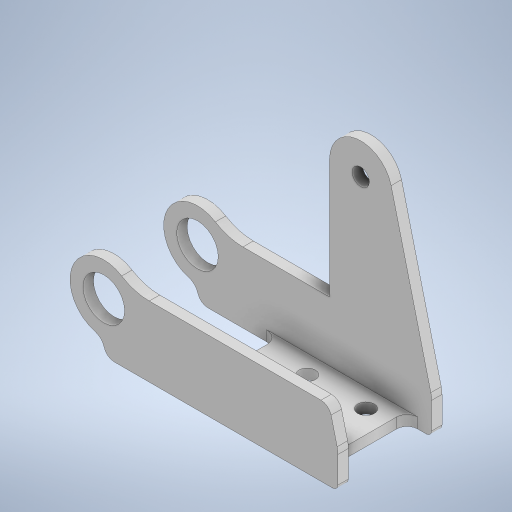
# Autodesk Inventor part: front joint
Saved by Autodesk Inventor 2023 (Build 270158000, 158)
## iProperties
Created: 2022-06-23
Part Number: front joint
Material: 一般
Document SubType Name: Modeling
Designer: 黃宇陽
Density: 1 g/cm^3
Appearance: 預設
Author: 黃宇陽
Autodesk Inventor part; units mm, degrees
ref_plane "YZ Plane" through (0, 0, 0) normal (1, 0, 0) x (0, 1, 0)
ref_plane "XZ Plane" through (0, 0, 0) normal (0, 1, 0) x (-1, 0, 0)
ref_plane "XY Plane" through (0, 0, 0) normal (0, 0, 1) x (1, 0, 0)
sketch "草圖1" plane through (0, 0, 0) normal (0, 0, 1) x (1, 0, 0)
  line L0 (0, 0) -> (-43, 0)
  line L1 (0, 0) -> (0, 6.7073)
  line L2 (0, 6.7073) -> (-1.691, 13.5)
  line L3 (-1.691, 13.5) -> (-36.2631, 13.5)
  arc A0 (-41.5549, 15.0149) -> (-36.2631, 13.5) centre (-36.2631, 23.5) ccw
  arc A1 (-41.5549, 15.0149) -> (-46.6885, 3.2242) centre (-44.9946, 9.4996) ccw
  arc A2 (-44.9289, 1.4714) -> (-46.6885, 3.2242) centre (-47.34, 0.8106) ccw
  arc A3 (-44.9289, 1.4714) -> (-43, 0) centre (-43, 2) ccw
  circle A4 centre (-44.9946, 9.4996) radius 4
  dimension "d0" = 43
  dimension "d1" = 13.5
  dimension "d2" = 10
  dimension "d3" = 2
  dimension "d6" = 2.5
  dimension "d7" = 6.5
  dimension "d8" = 4.899
  dimension "d9" = 2.426
  dimension "d10" = 7
  dimension "d11" = 6.7073
  dimension "d12" = 8
  constraints: 8 end point, 8 point on circle, 5 centre point, 5 tangent, 1 coincident, 1 horizontal, 1 perpendicular, 1 vertical
  measures "d0" distance of L0.start L0.end
  measures "d1" distance between parallel lines of L0 L3
  measures "d2" radius of A0
  measures "d3" radius of A3
  measures "d6" radius of A2
  measures "d7" radius of A1
  measures "d8" distance of L0.end A1.end
  measures "d9" distance of L0.end A2.start
  measures "d10" distance of L1.end L2.end
  measures "d11" distance from line of L0 L1.end
  measures "d12" diameter of A4
extrude "擠出1" add sketch "草圖1" along normal blind 20
sketch "草圖2" plane through (-36.2631, 13.5, 0) normal (0, 1, 0) x (1, 0, 0)
  line L0 (36.2631, 0) -> (36.2631, -20) construction
  line L1 (34.572, -20) -> (0, -20) projected
  line L2 (34.572, 0) -> (34.572, -20) projected
  arc A0 (31.5631, -16) -> (33.5631, -18) centre (33.5631, -16) ccw
  line L3 (31.5631, -16) -> (31.5631, -4)
  arc A1 (33.5631, -2) -> (31.5631, -4) centre (33.5631, -4) ccw
  line L4 (33.5631, -18) -> (4.5631, -18)
  line L5 (33.5631, -2) -> (4.5631, -2)
  arc A2 (4.5631, -18) -> (7.0631, -15.5) centre (4.5631, -15.5) ccw
  line L6 (7.0631, -15.5) -> (7.0631, -4.5)
  arc A3 (7.0631, -4.5) -> (4.5631, -2) centre (4.5631, -4.5) ccw
  circle A4 centre (27.2631, -14.4) radius 1.6
  line L7 (27.2631, -14.4) -> (27.2631, -5.6) construction
  circle A5 centre (27.2631, -5.6) radius 1.6
  line L8 (27.2631, -14.4) -> (15.9631, -14.4) construction
  line L9 (15.9631, -14.4) -> (15.9631, -5.6) construction
  circle A6 centre (15.9631, -14.4) radius 1.6
  circle A7 centre (15.9631, -5.6) radius 1.6
  circle A8 centre (10.8631, -10) radius 1.6
  line L10 (33.5631, -18) -> (36.2631, -18)
  line L11 (36.2631, 0) -> (36.2631, -20) projected
  line L12 (33.5631, -2) -> (36.2631, -2)
  line L13 (36.2631, -18) -> (36.2631, -2)
  line L14 (-15.2315, 0) -> (-15.2315, -20) projected
  line L15 (4.5631, -18) -> (-15.2315, -18)
  line L16 (4.5631, -2) -> (-15.2315, -2)
  line L17 (-15.2315, -18) -> (-15.2315, -2)
  dimension "d22" = 2
  dimension "d24" = 2
  dimension "d25" = 2
  dimension "d26" = 4.7
  dimension "d27" = 16
  dimension "d28" = 29
  dimension "d29" = 2.5
  dimension "d30" = 2.5
  dimension "d31" = 3.2
  dimension "d32" = 4.3
  dimension "d33" = 3.6
  dimension "d34" = 8.8
  dimension "d35" = 11.3
  dimension "d36" = 8.8
  dimension "d38" = 23.709
  dimension "d39" = 10
  constraints: 26 end point, 9 centre point, 8 point on circle, 7 tangent, 4 equal radius, 4 horizontal, 4 point on line, 4 vertical, 3 coincident, 3 perpendicular, 2 collinear, 1 parallel
  measures "d22" distance from line of L1 L4.start
  measures "d24" radius of A0
  measures "d25" radius of A1
  measures "d26" distance between parallel lines of L0 L3
  measures "d27" distance of L5.start L4.start
  measures "d28" distance of L4.start L4.end
  measures "d29" radius of A2
  measures "d30" radius of A3
  measures "d31" diameter of A4
  measures "d32" distance from line of L3 L7.start
  measures "d33" distance from line of L4 L7.start
  measures "d34" distance of L7.start L7.end
  measures "d35" distance of L7.start L8.end
  measures "d36" distance of L8.end L9.end
  measures "d38" distance from line of L2 A8.centre
  measures "d39" distance from line of L1 A8.centre
extrude "擠出2" cut sketch "草圖2" against normal blind 11.5 contours A1 L3 A0 L4 A2 L6 A3 L5 | A4 | A5 | A6 | A7 | A8
extrude "擠出3" cut sketch "草圖2" against normal through all contours A4 | A5 | A6 | A7 | A8
extrude "擠出4" cut sketch "草圖2" along normal through all both and the other way through all contours L12 L11 L10 L2 | L2 L10 A0 L3 A1 L12 | A3 L6 A2 L15 L14 L16
sketch "草圖3" plane through (0, 0, 0) normal (0, 0, -1) x (-1, 0, 0)
  line L0 (0, 6.7073) -> (0, 0) projected
  line L1 (0, 6.7073) -> (7.7777, 37.9495)
  line L2 (0, 6.7073) -> (1.691, 13.5) projected
  arc A0 (19.6, 36.5) -> (7.7777, 37.9495) centre (13.6, 36.5) ccw
  line L3 (19.6, 36.5) -> (19.6, 13.5)
  line L4 (19.6, 13.5) -> (0, 6.7073)
  line L5 (43, 0) -> (0, 0) projected
  circle A1 centre (13.6, 36.5) radius 1.65
  dimension "d46" = 36.5
  dimension "d47" = 6
  dimension "d48" = 23
  dimension "d49" = 3.3
  constraints: 6 end point, 2 centre point, 2 point on circle, 2 tangent, 1 coincident, 1 collinear, 1 vertical
  measures "d46" distance from line of L5 A0.centre
  measures "d47" radius of A0
  measures "d48" distance of L3.start L3.end
  measures "d49" diameter of A1
extrude "擠出5" add sketch "草圖3" against normal blind 2
fillet "圓角1" radius 1 2 edges at (0, 0, 19) (0, 0, 1)
fillet "圓角1" radius 5 2 edges at (0, 6.7073, 19) (0, 6.7073, 1)
fillet "圓角1" radius 2 1 edges at (-1.691, 13.5, 19)
